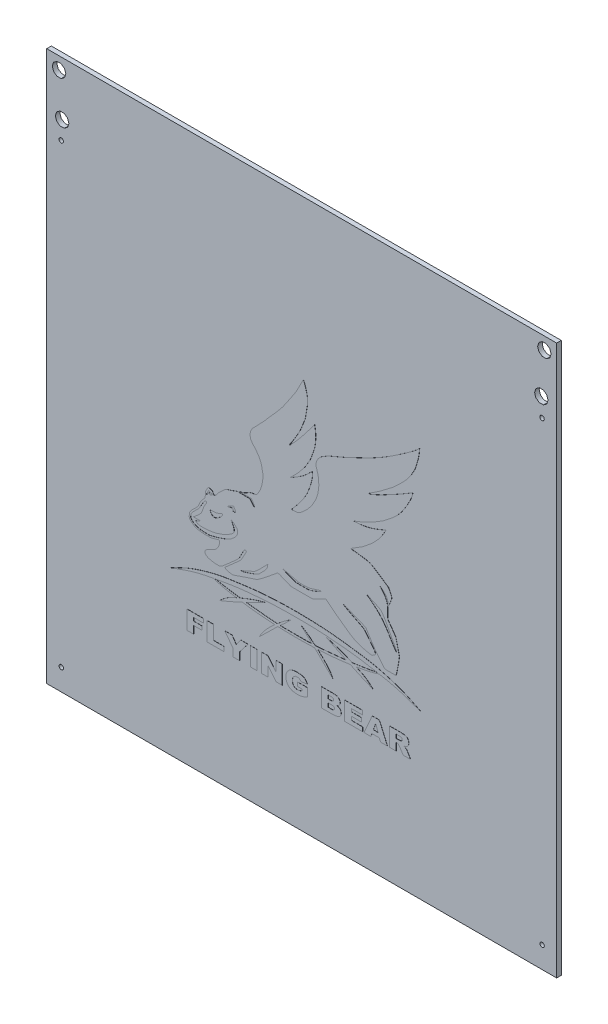
# Autodesk Inventor part: боковая  панель
Saved by Autodesk Inventor 2017 (Build 210142000, 142)
## iProperties
Part Number: боковая  панель
Material: Типовые
Document SubType Name: Modeling
Designer: Max
Mass: 356.832 g
Surface Area: 2420.3 cm^2
Volume: 356.832 cm^3
Density: 1 g/cm^3
Appearance: Чугун серый
Author: Max
Autodesk Inventor part; units mm, degrees
(part 1 of 2)
ref_plane "YZ Plane" through (0, 0, 0) normal (1, 0, 0) x (0, 1, 0)
ref_plane "XZ Plane" through (0, 0, 0) normal (0, 1, 0) x (-1, 0, 0)
ref_plane "XY Plane" through (0, 0, 0) normal (0, 0, 1) x (1, 0, 0)
sketch "Эскиз1" plane through (0, 0, 0) normal (0, 0, 1) x (1, 0, 0)
  circle A0 centre (8.5, 9) radius 1.5 projected
  circle A1 centre (8.5, 306) radius 1.5 projected
  circle A2 centre (-304.5, 306) radius 1.5 projected
  circle A3 centre (-304.5, 9) radius 1.5 projected
  line L0 (-314, 353) -> (18, 353)
  line L1 (18, 353) -> (18, -5)
  line L2 (18, -5) -> (-314, -5)
  line L3 (-314, -5) -> (-314, 353)
  circle A4 centre (10, 345) radius 4.4
  circle A5 centre (8, 318) radius 4.4
  circle A6 centre (-306, 345) radius 4.4
  circle A7 centre (-304, 318) radius 4.4
  point P0 (0, 0)
  dimension "d0" = 297
  dimension "d1" = 313
  dimension "d2" = 9.5
  dimension "d3" = 9.5
  dimension "d4" = 332
  dimension "d5" = 9.5
  dimension "d6" = 358
  dimension "d7" = 14
  dimension "d8" = 47
  dimension "d26" = 8
  dimension "d27" = 8
  dimension "d28" = 10
  dimension "d29" = 35
  dimension "d30" = 8
  dimension "d31" = 35
  dimension "d32" = 10
  dimension "d33" = 8
  dimension "d34" = 8.8
  dimension "d35" = 8.8
  dimension "d36" = 8.8
  dimension "d37" = 8.8
  constraints: 8 end point, 4 centre point, 2 parallel, 1 horizontal, 1 perpendicular
  measures "d0" distance of A0.centre A1.centre
  measures "d1" distance of A0.centre A3.centre
  measures "d2" distance from line of L1 A0.centre
  measures "d3" distance from line of L1 A1.centre
  measures "d4" distance between parallel lines of L1 L3
  measures "d5" distance from line of A3.centre L3
  measures "d6" distance between parallel lines of L0 L2
  measures "d7" distance from line of A3.centre L2
  measures "d8" distance from line of L0 A2.centre
  measures "d26" distance from line of L1 A4.centre
  measures "d27" distance from line of A4.centre L0
  measures "d28" distance from line of L1 A5.centre
  measures "d29" distance from line of L0 A5.centre
  measures "d30" distance from line of L0 A6.centre
  measures "d31" distance from line of A7.centre L0
  measures "d32" horizontal distance of L0.start A7.centre
  measures "d33" horizontal distance of A6.centre L0.start
  measures "d34" diameter of A6
  measures "d35" diameter of A7
  measures "d36" diameter of A4
  measures "d37" diameter of A5
extrude "Выдавливание1" add sketch "Эскиз1" along normal blind 3
sketch "Эскиз2" plane through (0, 0, 3) normal (0, 0, 1) x (1, 0, 0)
  line L0 (-180.2045, 205.6908) -> (-177.0361, 208.9639) construction
  line L1 (-177.0361, 208.9639) -> (-173.0672, 213.1037) construction
  line L2 (-173.0672, 213.1037) -> (-170.4432, 215.9574) construction
  line L3 (-170.4432, 215.9574) -> (-168.8687, 218.0566) construction
  line L4 (-168.8687, 218.0566) -> (-164.9525, 222.1283) construction
  line L5 (-164.9525, 222.1283) -> (-161.4603, 226.3362) construction
  line L6 (-161.4603, 226.3362) -> (-160.288, 227.7676) construction
  line L7 (-160.288, 227.7676) -> (-152.6607, 239.1023) construction
  line L8 (-152.6607, 239.1023) -> (-151.6323, 240.6673) construction
  line L9 (-151.6323, 240.6673) -> (-149.9316, 243.8361) construction
  line L10 (-149.9316, 243.8361) -> (-148.3507, 246.9727) construction
  line L11 (-148.3507, 246.9727) -> (-146.851, 249.9512) construction
  line L12 (-146.851, 249.9512) -> (-146.8254, 250.015) construction
  line L13 (-146.8254, 250.015) -> (-146.8254, 249.9575) construction
  line L14 (-146.8254, 249.9575) -> (-146.0075, 248.3799) construction
  line L15 (-146.0075, 248.3799) -> (-144.426, 243.2509) construction
  line L16 (-144.426, 243.2509) -> (-144.0276, 240.6093) construction
  line L17 (-144.0276, 240.6093) -> (-144.0276, 237.8628) construction
  line L18 (-144.0276, 237.8628) -> (-145.0701, 229.6994) construction
  line L19 (-145.0701, 229.6994) -> (-146.4307, 225.9017) construction
  line L20 (-146.4307, 225.9017) -> (-149.1507, 219.4923) construction
  line L21 (-149.1507, 219.4923) -> (-151.6499, 215.3156) construction
  line L22 (-151.6499, 215.3156) -> (-154.3887, 211.0362) construction
  line L23 (-154.3887, 211.0362) -> (-155.1076, 209.9749) construction
  line L24 (-155.1076, 209.9749) -> (-156.1304, 208.4939) construction
  line L25 (-156.1304, 208.4939) -> (-155.9009, 208.6294) construction
  line L26 (-155.9009, 208.6294) -> (-155.5783, 208.8301) construction
  line L27 (-155.5783, 208.8301) -> (-154.5963, 209.615) construction
  line L28 (-154.5963, 209.615) -> (-150.9546, 213.5612) construction
  line L29 (-150.9546, 213.5612) -> (-145.5874, 220.0786) construction
  line L30 (-145.5874, 220.0786) -> (-139.5565, 228.2444) construction
  line L31 (-139.5565, 228.2444) -> (-139.4969, 228.3364) construction
  line L32 (-139.4969, 228.3364) -> (-139.5299, 228.2418) construction
  line L33 (-139.5299, 228.2418) -> (-139.3563, 227.561) construction
  line L34 (-139.3563, 227.561) -> (-138.9367, 225.0891) construction
  line L35 (-138.9367, 225.0891) -> (-138.5378, 221.4685) construction
  line L36 (-138.5378, 221.4685) -> (-139.0937, 215.6761) construction
  line L37 (-139.0937, 215.6761) -> (-140.9097, 209.7093) construction
  line L38 (-140.9097, 209.7093) -> (-143.5781, 204.4836) construction
  line L39 (-143.5781, 204.4836) -> (-146.543, 199.8881) construction
  line L40 (-146.543, 199.8881) -> (-150.7936, 195.0629) construction
  line L41 (-150.7936, 195.0629) -> (-152.871, 193.083) construction
  line L42 (-152.871, 193.083) -> (-154.5999, 191.4239) construction
  line L43 (-154.5999, 191.4239) -> (-155.5201, 190.4339) construction
  line L44 (-155.5201, 190.4339) -> (-155.5742, 190.3528) construction
  line L45 (-155.5742, 190.3528) -> (-155.4326, 190.4314) construction
  line L46 (-155.4326, 190.4314) -> (-153.8538, 191.4333) construction
  line L47 (-153.8538, 191.4333) -> (-152.2645, 192.2568) construction
  line L48 (-152.2645, 192.2568) -> (-149.2402, 194.1507) construction
  line L49 (-149.2402, 194.1507) -> (-146.2078, 196.1384) construction
  line L50 (-146.2078, 196.1384) -> (-144.4494, 197.8457) construction
  line L51 (-144.4494, 197.8457) -> (-142.5127, 199.706) construction
  line L52 (-142.5127, 199.706) -> (-141.1876, 201.0821) construction
  line L53 (-141.1876, 201.0821) -> (-141.1211, 201.1736) construction
  line L54 (-141.1211, 201.1736) -> (-141.1521, 201.0592) construction
  line L55 (-141.1521, 201.0592) -> (-140.789, 198.921) construction
  line L56 (-140.789, 198.921) -> (-141.0832, 196.2734) construction
  line L57 (-141.0832, 196.2734) -> (-143.5783, 187.7744) construction
  line L58 (-143.5783, 187.7744) -> (-147.4823, 181.1681) construction
  line L59 (-147.4823, 181.1681) -> (-154.6365, 172.9333) construction
  line L60 (-154.6365, 172.9333) -> (-154.6413, 172.9279) construction
  line L61 (-154.6413, 172.9279) -> (-154.6261, 172.9325) construction
  line L62 (-154.6261, 172.9325) -> (-150.5488, 173.1303) construction
  line L63 (-150.5488, 173.1303) -> (-150.5023, 173.1303) construction
  line L64 (-150.5023, 173.1303) -> (-150.4241, 173.1753) construction
  line L65 (-150.4241, 173.1753) -> (-148.6376, 174.0969) construction
  line L66 (-148.6376, 174.0969) -> (-145.9899, 176.3194) construction
  line L67 (-145.9899, 176.3194) -> (-143.6414, 178.7272) construction
  line L68 (-143.6414, 178.7272) -> (-141.2139, 181.648) construction
  line L69 (-141.2139, 181.648) -> (-138.637, 186.2308) construction
  line L70 (-138.637, 186.2308) -> (-137.7784, 188.5813) construction
  line L71 (-137.7784, 188.5813) -> (-136.7423, 192.9865) construction
  line L72 (-136.7423, 192.9865) -> (-136.7423, 195.346) construction
  line L73 (-136.7423, 195.346) -> (-136.7423, 199.308) construction
  line L74 (-136.7423, 199.308) -> (-137.351, 201.832) construction
  line L75 (-137.351, 201.832) -> (-137.9585, 203.1815) construction
  line L76 (-137.9585, 203.1815) -> (-138.5823, 204.6492) construction
  line L77 (-138.5823, 204.6492) -> (-138.7474, 205.6908) construction
  line L78 (-138.7474, 205.6908) -> (-138.5929, 207.7385) construction
  line L79 (-138.5929, 207.7385) -> (-137.7581, 209.4958) construction
  line L80 (-137.7581, 209.4958) -> (-136.7322, 211.0337) construction
  line L81 (-136.7322, 211.0337) -> (-134.1061, 213.2212) construction
  line L82 (-134.1061, 213.2212) -> (-131.0548, 214.9609) construction
  line L83 (-131.0548, 214.9609) -> (-125.9426, 217.1289) construction
  line L84 (-125.9426, 217.1289) -> (-120.429, 219.2434) construction
  line L85 (-120.429, 219.2434) -> (-111.0683, 223.8533) construction
  line L86 (-111.0683, 223.8533) -> (-101.1893, 228.475) construction
  line L87 (-101.1893, 228.475) -> (-91.9176, 233.9051) construction
  line L88 (-91.9176, 233.9051) -> (-86.9496, 237.2556) construction
  line L89 (-86.9496, 237.2556) -> (-76.65, 244.2967) construction
  line L90 (-76.65, 244.2967) -> (-73.4984, 246.8715) construction
  line L91 (-73.4984, 246.8715) -> (-71.8505, 248.334) construction
  line L92 (-71.8505, 248.334) -> (-71.1089, 249.0344) construction
  line L93 (-71.1089, 249.0344) -> (-71.0317, 249.0344) construction
  line L94 (-71.0317, 249.0344) -> (-71.2255, 248.5055) construction
  line L95 (-71.2255, 248.5055) -> (-71.2255, 246.9556) construction
  line L96 (-71.2255, 246.9556) -> (-71.9453, 242.6946) construction
  line L97 (-71.9453, 242.6946) -> (-73.4931, 236.8072) construction
  line L98 (-73.4931, 236.8072) -> (-75.2923, 233.1849) construction
  line L99 (-75.2923, 233.1849) -> (-78.2429, 228.7711) construction
  line L100 (-78.2429, 228.7711) -> (-80.9056, 225.6046) construction
  line L101 (-80.9056, 225.6046) -> (-88.7168, 218.0744) construction
  line L102 (-88.7168, 218.0744) -> (-93.9004, 214.1054) construction
  line L103 (-93.9004, 214.1054) -> (-101.4492, 208.9934) construction
  line L104 (-101.4492, 208.9934) -> (-104.0858, 207.4669) construction
  line L105 (-104.0858, 207.4669) -> (-104.0858, 207.3813) construction
  line L106 (-104.0858, 207.3813) -> (-103.6066, 207.0724) construction
  line L107 (-103.6066, 207.0724) -> (-102.7892, 207.2333) construction
  line L108 (-102.7892, 207.2333) -> (-96.5868, 210.0566) construction
  line L109 (-96.5868, 210.0566) -> (-85.8931, 215.7161) construction
  line L110 (-85.8931, 215.7161) -> (-79.7646, 219.312) construction
  line L111 (-79.7646, 219.312) -> (-75.6998, 221.7509) construction
  line L112 (-75.6998, 221.7509) -> (-75.5621, 221.8387) construction
  line L113 (-75.5621, 221.8387) -> (-75.5621, 221.3223) construction
  line L114 (-75.5621, 221.3223) -> (-77.0245, 216.3152) construction
  line L115 (-77.0245, 216.3152) -> (-82.7085, 207.0734) construction
  line L116 (-82.7085, 207.0734) -> (-86.2044, 203.347) construction
  line L117 (-86.2044, 203.347) -> (-91.7733, 198.4009) construction
  line L118 (-91.7733, 198.4009) -> (-96.3023, 195.3488) construction
  line L119 (-96.3023, 195.3488) -> (-102.062, 191.8536) construction
  line L120 (-102.062, 191.8536) -> (-107.7725, 189.2445) construction
  line L121 (-107.7725, 189.2445) -> (-112.1538, 187.3246) construction
  line L122 (-112.1538, 187.3246) -> (-113.8768, 186.98) construction
  line L123 (-113.8768, 186.98) -> (-114.0125, 186.7136) construction
  line L124 (-114.0125, 186.7136) -> (-113.6533, 186.5708) construction
  line L125 (-113.6533, 186.5708) -> (-107.5747, 186.9569) construction
  line L126 (-107.5747, 186.9569) -> (-101.6244, 188.5451) construction
  line L127 (-101.6244, 188.5451) -> (-97.9782, 189.9544) construction
  line L128 (-97.9782, 189.9544) -> (-93.3535, 191.865) construction
  line L129 (-93.3535, 191.865) -> (-92.8714, 192.0615) construction
  line L130 (-92.8714, 192.0615) -> (-93.1602, 191.852) construction
  line L131 (-93.1602, 191.852) -> (-93.9679, 190.2952) construction
  line L132 (-93.9679, 190.2952) -> (-96.2883, 186.5339) construction
  line L133 (-96.2883, 186.5339) -> (-98.0685, 184.2257) construction
  line L134 (-98.0685, 184.2257) -> (-101.6348, 180.439) construction
  line L135 (-101.6348, 180.439) -> (-106.2734, 176.3065) construction
  line L136 (-106.2734, 176.3065) -> (-110.5464, 173.5515) construction
  line L137 (-110.5464, 173.5515) -> (-114.6789, 171.1058) construction
  line L138 (-114.6789, 171.1058) -> (-116.1126, 170.2062) construction
  line L139 (-116.1126, 170.2062) -> (-116.219, 170.0286) construction
  line L140 (-116.219, 170.0286) -> (-114.5586, 170.0286) construction
  line L141 (-114.5586, 170.0286) -> (-110.6732, 169.621) construction
  line L142 (-110.6732, 169.621) -> (-104.7271, 168.6199) construction
  line L143 (-104.7271, 168.6199) -> (-103.1534, 168.6199) construction
  line L144 (-103.1534, 168.6199) -> (-91.4021, 160.5335) construction
  line L145 (-91.4021, 160.5335) -> (-91.3533, 160.4774) construction
  line L146 (-91.3533, 160.4774) -> (-91.1816, 160.134) construction
  line L147 (-91.1816, 160.134) -> (-89.1661, 156.0741) construction
  line L148 (-89.1661, 156.0741) -> (-89.1661, 155.5737) construction
  line L149 (-89.1661, 155.5737) -> (-89.5681, 154.2932) construction
  line L150 (-89.5681, 154.2932) -> (-90.5395, 151.4784) construction
  line L151 (-90.5395, 151.4784) -> (-91.257, 150.209) construction
  line L152 (-91.257, 150.209) -> (-91.566, 150.1317) construction
  line L153 (-91.566, 150.1317) -> (-91.566, 150.2531) construction
  line L154 (-91.566, 150.2531) -> (-91.566, 150.7278) construction
  line L155 (-91.566, 150.7278) -> (-91.6764, 152.0082) construction
  line L156 (-91.6764, 152.0082) -> (-91.9413, 153.1783) construction
  line L157 (-91.9413, 153.1783) -> (-92.6368, 155.088) construction
  line L158 (-92.6368, 155.088) -> (-94.3256, 156.6333) construction
  line L159 (-94.3256, 156.6333) -> (-95.9262, 158.0242) construction
  line L160 (-95.9262, 158.0242) -> (-96.6768, 158.3222) construction
  line L161 (-96.6768, 158.3222) -> (-96.9749, 158.3995) construction
  line L162 (-96.9749, 158.3995) -> (-96.8701, 158.3475) construction
  line L163 (-96.8701, 158.3475) -> (-96.2956, 157.8766) construction
  line L164 (-96.2956, 157.8766) -> (-94.9273, 156.285) construction
  line L165 (-94.9273, 156.285) -> (-93.124, 153.9456) construction
  line L166 (-93.124, 153.9456) -> (-92.5148, 152.3129) construction
  line L167 (-92.5148, 152.3129) -> (-91.9299, 149.9735) construction
  line L168 (-91.9299, 149.9735) -> (-91.9299, 148.9594) construction
  line L169 (-91.9299, 148.9594) -> (-91.9299, 142.9463) construction
  line L170 (-91.9299, 142.9463) -> (-91.9299, 142.2235) construction
  line L171 (-91.9299, 142.2235) -> (-90.4742, 140.5124) construction
  line L172 (-90.4742, 140.5124) -> (-86.5347, 134.8618) construction
  line L173 (-86.5347, 134.8618) -> (-86.3052, 134.3183) construction
  line L174 (-86.3052, 134.3183) -> (-86.3052, 133.0505) construction
  line L175 (-86.3052, 133.0505) -> (-84.3022, 125.647) construction
  line L176 (-84.3022, 125.647) -> (-84.3022, 124.6994) construction
  line L177 (-84.3022, 124.6994) -> (-84.5184, 122.8172) construction
  line L178 (-84.5184, 122.8172) -> (-86.3367, 113.3336) construction
  line L179 (-86.3367, 113.3336) -> (-86.5078, 113.3336) construction
  line L180 (-86.5078, 113.3336) -> (-87.2901, 113.3336) construction
  line L181 (-87.2901, 113.3336) -> (-93.4748, 113.3336) construction
  line L182 (-93.4748, 113.3336) -> (-94.0214, 113.3336) construction
  line L183 (-94.0214, 113.3336) -> (-94.9467, 114.9961) construction
  line L184 (-94.9467, 114.9961) -> (-98.9456, 119.3916) construction
  line L185 (-98.9456, 119.3916) -> (-100.0032, 120.9448) construction
  line L186 (-100.0032, 120.9448) -> (-106.018, 130.2315) construction
  line L187 (-106.018, 130.2315) -> (-106.215, 130.694) construction
  line L188 (-106.215, 130.694) -> (-106.6783, 130.8203) construction
  line L189 (-106.6783, 130.8203) -> (-120.5865, 136.5083) construction
  line L190 (-120.5865, 136.5083) -> (-120.6842, 136.5083) construction
  line L191 (-120.6842, 136.5083) -> (-120.6842, 135.7899) construction
  line L192 (-120.6842, 135.7899) -> (-107.7997, 129.5862) construction
  line L193 (-107.7997, 129.5862) -> (-107.1982, 129.0639) construction
  line L194 (-107.1982, 129.0639) -> (-106.0151, 127.5405) construction
  line L195 (-106.0151, 127.5405) -> (-101.2131, 121.3926) construction
  line L196 (-101.2131, 121.3926) -> (-99.7156, 119.3405) construction
  line L197 (-99.7156, 119.3405) -> (-99.7156, 118.1853) construction
  line L198 (-99.7156, 118.1853) -> (-101.9371, 116.8524) construction
  line L199 (-101.9371, 116.8524) -> (-103.5365, 116.8524) construction
  line L200 (-103.5365, 116.8524) -> (-107.4464, 117.9484) construction
  line L201 (-107.4464, 117.9484) -> (-112.9293, 119.2821) construction
  line L202 (-112.9293, 119.2821) -> (-117.2673, 122.3561) construction
  line L203 (-117.2673, 122.3561) -> (-125.6526, 128.3292) construction
  line L204 (-125.6526, 128.3292) -> (-132.3149, 133.728) construction
  line L205 (-132.3149, 133.728) -> (-132.126, 133.8212) construction
  line L206 (-132.126, 133.8212) -> (-132.8175, 133.2753) construction
  line L207 (-132.8175, 133.2753) -> (-140.6236, 129.3632) construction
  line L208 (-140.6236, 129.3632) -> (-140.9553, 129.3632) construction
  line L209 (-140.9553, 129.3632) -> (-142.7265, 129.3632) construction
  line L210 (-142.7265, 129.3632) -> (-154.9526, 129.3632) construction
  line L211 (-154.9526, 129.3632) -> (-155.1733, 129.4132) construction
  line L212 (-155.1733, 129.4132) -> (-155.4392, 129.6496) construction
  line L213 (-155.4392, 129.6496) -> (-163.3327, 132.864) construction
  line L214 (-163.3327, 132.864) -> (-163.5864, 132.864) construction
  line L215 (-163.5864, 132.864) -> (-164.5688, 131.6844) construction
  line L216 (-164.5688, 131.6844) -> (-176.3163, 122.4788) construction
  line L217 (-176.3163, 122.4788) -> (-176.8534, 122.1588) construction
  line L218 (-176.8534, 122.1588) -> (-182.8586, 120.3906) construction
  line L219 (-182.8586, 120.3906) -> (-192.5336, 116.921) construction
  line L220 (-192.5336, 116.921) -> (-193.8347, 116.7208) construction
  line L221 (-193.8347, 116.7208) -> (-195.9031, 117.4548) construction
  line L222 (-195.9031, 117.4548) -> (-198.1717, 118.4556) construction
  line L223 (-198.1717, 118.4556) -> (-198.1717, 118.5559) construction
  line L224 (-198.1717, 118.5559) -> (-197.5373, 118.8968) construction
  line L225 (-197.5373, 118.8968) -> (-187.5242, 127.8743) construction
  line L226 (-187.5242, 127.8743) -> (-187.343, 127.9999) construction
  line L227 (-187.343, 127.9999) -> (-187.0311, 128.8156) construction
  line L228 (-187.0311, 128.8156) -> (-183.7764, 134.5353) construction
  line L229 (-183.7764, 134.5353) -> (-183.7764, 134.6318) construction
  line L230 (-183.7764, 134.6318) -> (-185.0783, 135.1622) construction
  line L231 (-185.0783, 135.1622) -> (-185.3677, 134.8384) construction
  line L232 (-185.3677, 134.8384) -> (-188.4981, 128.4994) construction
  line L233 (-188.4981, 128.4994) -> (-188.8328, 127.9639) construction
  line L234 (-188.8328, 127.9639) -> (-200.3103, 117.8026) construction
  line L235 (-200.3103, 117.8026) -> (-201.0177, 117.5182) construction
  line L236 (-201.0177, 117.5182) -> (-203.6469, 117.5182) construction
  line L237 (-203.6469, 117.5182) -> (-206.0855, 117.8611) construction
  line L238 (-206.0855, 117.8611) -> (-209.5599, 118.534) construction
  line L239 (-209.5599, 118.534) -> (-211.0538, 120.2854) construction
  line L240 (-211.0538, 120.2854) -> (-211.0538, 121.2384) construction
  line L241 (-211.0538, 121.2384) -> (-210.4357, 122.3717) construction
  line L242 (-210.4357, 122.3717) -> (-208.0146, 123.9686) construction
  line L243 (-208.0146, 123.9686) -> (-206.0828, 124.4322) construction
  line L244 (-206.0828, 124.4322) -> (-203.7647, 125.8231) construction
  line L245 (-203.7647, 125.8231) -> (-203.4299, 126.1837) construction
  line L246 (-203.4299, 126.1837) -> (-202.0648, 127.9351) construction
  line L247 (-202.0648, 127.9351) -> (-201.5497, 129.6865) construction
  line L248 (-201.5497, 129.6865) -> (-201.3054, 130.6523) construction
  line L249 (-201.3054, 130.6523) -> (-201.6177, 132.2504) construction
  line L250 (-201.6177, 132.2504) -> (-201.783, 132.2504) construction
  line L251 (-201.783, 132.2504) -> (-202.7749, 131.9381) construction
  line L252 (-202.7749, 131.9381) -> (-204.7771, 131.2401) construction
  line L253 (-204.7771, 131.2401) -> (-207.9548, 130.487) construction
  line L254 (-207.9548, 130.487) -> (-210.9579, 130.6932) construction
  line L255 (-210.9579, 130.6932) -> (-215.2456, 131.0336) construction
  line L256 (-215.2456, 131.0336) -> (-216.2846, 131.323) construction
  line L257 (-216.2846, 131.323) -> (-218.5042, 132.1029) construction
  line L258 (-218.5042, 132.1029) -> (-220.9938, 134.2925) construction
  line L259 (-220.9938, 134.2925) -> (-221.2338, 135.6423) construction
  line L260 (-221.2338, 135.6423) -> (-221.2338, 137.742) construction
  line L261 (-221.2338, 137.742) -> (-220.1239, 139.6916) construction
  line L262 (-220.1239, 139.6916) -> (-218.5386, 141.0887) construction
  line L263 (-218.5386, 141.0887) -> (-216.5319, 143.019) construction
  line L264 (-216.5319, 143.019) -> (-215.5189, 143.8026) construction
  line L265 (-215.5189, 143.8026) -> (-214.1688, 146.7968) construction
  line L266 (-214.1688, 146.7968) -> (-213.4971, 148.6055) construction
  line L267 (-213.4971, 148.6055) -> (-211.921, 150.0782) construction
  line L268 (-211.921, 150.0782) -> (-210.7977, 151.1461) construction
  line L269 (-210.7977, 151.1461) -> (-210.573, 151.8599) construction
  line L270 (-210.573, 151.8599) -> (-210.7321, 154.5841) construction
  line L271 (-210.7321, 154.5841) -> (-210.5325, 155.5529) construction
  line L272 (-210.5325, 155.5529) -> (-209.9889, 156.8112) construction
  line L273 (-209.9889, 156.8112) -> (-209.0662, 157.9485) construction
  line L274 (-209.0662, 157.9485) -> (-208.6799, 158.485) construction
  line L275 (-208.6799, 158.485) -> (-206.6842, 158.2275) construction
  line L276 (-206.6842, 158.2275) -> (-205.7186, 157.2833) construction
  line L277 (-205.7186, 157.2833) -> (-205.3324, 156.3176) construction
  line L278 (-205.3324, 156.3176) -> (-205.3324, 155.7812) construction
  line L279 (-205.3324, 155.7812) -> (-204.7499, 155.7812) construction
  line L280 (-204.7499, 155.7812) -> (-203.9962, 156.222) construction
  line L281 (-203.9962, 156.222) -> (-203.2597, 156.7873) construction
  line L282 (-203.2597, 156.7873) -> (-202.8979, 158.1961) construction
  line L283 (-202.8979, 158.1961) -> (-197.8496, 162.6422) construction
  line L284 (-197.8496, 162.6422) -> (-197.2244, 163.0822) construction
  line L285 (-197.2244, 163.0822) -> (-195.8581, 163.3369) construction
  line L286 (-195.8581, 163.3369) -> (-192.1429, 164.6422) construction
  line L287 (-192.1429, 164.6422) -> (-190.165, 165.3816) construction
  line L288 (-190.165, 165.3816) -> (-189.592, 165.5664) construction
  line L289 (-189.592, 165.5664) -> (-189.592, 165.4643) construction
  line L290 (-189.592, 165.4643) -> (-181.4929, 165.4643) construction
  line L291 (-181.4929, 165.4643) -> (-181.4186, 165.3756) construction
  line L292 (-181.4186, 165.3756) -> (-180.8085, 164.4859) construction
  line L293 (-180.8085, 164.4859) -> (-179.2071, 162.3253) construction
  line L294 (-179.2071, 162.3253) -> (-178.9159, 162.2122) construction
  line L295 (-178.9159, 162.2122) -> (-178.6217, 162.3643) construction
  line L296 (-178.6217, 162.3643) -> (-178.6826, 162.4252) construction
  line L297 (-178.6826, 162.4252) -> (-178.6826, 163.1963) construction
  line L298 (-178.6826, 163.1963) -> (-180.6203, 166.1181) construction
  line L299 (-180.6203, 166.1181) -> (-180.7015, 166.1181) construction
  line L300 (-180.7015, 166.1181) -> (-181.3406, 166.0572) construction
  line L301 (-181.3406, 166.0572) -> (-188.5602, 166.0572) construction
  line L302 (-188.5602, 166.0572) -> (-188.5291, 166.0841) construction
  line L303 (-188.5291, 166.0841) -> (-188.3128, 166.1085) construction
  line L304 (-188.3128, 166.1085) -> (-187.054, 166.3579) construction
  line L305 (-187.054, 166.3579) -> (-184.878, 166.9958) construction
  line L306 (-184.878, 166.9958) -> (-181.1411, 169.1807) construction
  line L307 (-181.1411, 169.1807) -> (-180.4894, 169.5066) construction
  line L308 (-180.4894, 169.5066) -> (-179.4678, 169.4127) construction
  line L309 (-179.4678, 169.4127) -> (-178.1345, 169.4425) construction
  line L310 (-178.1345, 169.4425) -> (-177.6022, 169.6366) construction
  line L311 (-177.6022, 169.6366) -> (-176.6134, 170.4786) construction
  line L312 (-176.6134, 170.4786) -> (-175.3808, 172.823) construction
  line L313 (-175.3808, 172.823) -> (-174.1929, 175.2387) construction
  line L314 (-174.1929, 175.2387) -> (-173.6413, 177.7553) construction
  line L315 (-173.6413, 177.7553) -> (-173.4172, 179.0825) construction
  line L316 (-173.4172, 179.0825) -> (-172.913, 182.4907) construction
  line L317 (-172.913, 182.4907) -> (-173.5125, 186.8632) construction
  line L318 (-173.5125, 186.8632) -> (-174.6056, 190.1425) construction
  line L319 (-174.6056, 190.1425) -> (-175.7692, 192.4698) construction
  line L320 (-175.7692, 192.4698) -> (-177.6734, 195.2202) construction
  line L321 (-177.6734, 195.2202) -> (-179.4012, 196.7718) construction
  line L322 (-179.4012, 196.7718) -> (-180.6411, 198.1746) construction
  line L323 (-180.6411, 198.1746) -> (-181.3601, 199.7249) construction
  line L324 (-181.3601, 199.7249) -> (-181.6297, 201.3426) construction
  line L325 (-181.6297, 201.3426) -> (-181.4275, 202.9153) construction
  line L326 (-181.4275, 202.9153) -> (-181.1129, 204.4206) construction
  line L327 (-181.1129, 204.4206) -> (-180.6636, 205.1396) construction
  line L328 (-180.6636, 205.1396) -> (-180.2045, 205.6908) construction
  spline S0 degree 4 poles (-180.2045, 205.6908) (-177.0361, 208.9639) (-173.0672, 213.1037) (-170.4432, 215.9574) (-168.8687, 218.0566) (-164.9525, 222.1283) (-161.4603, 226.3362) (-160.288, 227.7676) (-152.6607, 239.1023) (-151.6323, 240.6673) (-149.9316, 243.8361) (-148.3507, 246.9727) (-146.851, 249.9512) (-146.8254, 250.015) (-146.8254, 249.9575) (-146.0075, 248.3799) (-144.426, 243.2509) (-144.0276, 240.6093) (-144.0276, 237.8628) (-145.0701, 229.6994) (-146.4307, 225.9017) (-149.1507, 219.4923) (-151.6499, 215.3156) (-154.3887, 211.0362) (-155.1076, 209.9749) (-156.1304, 208.4939) (-155.9009, 208.6294) (-155.5783, 208.8301) (-154.5963, 209.615) (-150.9546, 213.5612) (-145.5874, 220.0786) (-139.5565, 228.2444) (-139.4969, 228.3364) (-139.5299, 228.2418) (-139.3563, 227.561) (-138.9367, 225.0891) (-138.5378, 221.4685) (-139.0937, 215.6761) (-140.9097, 209.7093) (-143.5781, 204.4836) (-146.543, 199.8881) (-150.7936, 195.0629) (-152.871, 193.083) (-154.5999, 191.4239) (-155.5201, 190.4339) (-155.5742, 190.3528) (-155.4326, 190.4314) (-153.8538, 191.4333) (-152.2645, 192.2568) (-149.2402, 194.1507) (-146.2078, 196.1384) (-144.4494, 197.8457) (-142.5127, 199.706) (-141.1876, 201.0821) (-141.1211, 201.1736) (-141.1521, 201.0592) (-140.789, 198.921) (-141.0832, 196.2734) (-143.5783, 187.7744) (-147.4823, 181.1681) (-154.6365, 172.9333) (-154.6413, 172.9279) (-154.6261, 172.9325) (-150.5488, 173.1303) (-150.5023, 173.1303) (-150.4241, 173.1753) (-148.6376, 174.0969) (-145.9899, 176.3194) (-143.6414, 178.7272) (-141.2139, 181.648) (-138.637, 186.2308) (-137.7784, 188.5813) (-136.7423, 192.9865) (-136.7423, 195.346) (-136.7423, 199.308) (-137.351, 201.832) (-137.9585, 203.1815) (-138.5823, 204.6492) (-138.7474, 205.6908) (-138.5929, 207.7385) (-137.7581, 209.4958) (-136.7322, 211.0337) (-134.1061, 213.2212) (-131.0548, 214.9609) (-125.9426, 217.1289) (-120.429, 219.2434) (-111.0683, 223.8533) (-101.1893, 228.475) (-91.9176, 233.9051) (-86.9496, 237.2556) (-76.65, 244.2967) (-73.4984, 246.8715) (-71.8505, 248.334) (-71.1089, 249.0344) (-71.0317, 249.0344) (-71.2255, 248.5055) (-71.2255, 246.9556) (-71.9453, 242.6946) (-73.4931, 236.8072) (-75.2923, 233.1849) (-78.2429, 228.7711) (-80.9056, 225.6046) (-88.7168, 218.0744) (-93.9004, 214.1054) (-101.4492, 208.9934) (-104.0858, 207.4669) (-104.0858, 207.3813) (-103.6066, 207.0724) (-102.7892, 207.2333) (-96.5868, 210.0566) (-85.8931, 215.7161) (-79.7646, 219.312) (-75.6998, 221.7509) (-75.5621, 221.8387) (-75.5621, 221.3223) (-77.0245, 216.3152) (-82.7085, 207.0734) (-86.2044, 203.347) (-91.7733, 198.4009) (-96.3023, 195.3488) (-102.062, 191.8536) (-107.7725, 189.2445) (-112.1538, 187.3246) (-113.8768, 186.98) (-114.0125, 186.7136) (-113.6533, 186.5708) (-107.5747, 186.9569) (-101.6244, 188.5451) (-97.9782, 189.9544) (-93.3535, 191.865) (-92.8714, 192.0615) (-93.1602, 191.852) (-93.9679, 190.2952) (-96.2883, 186.5339) (-98.0685, 184.2257) (-101.6348, 180.439) (-106.2734, 176.3065) (-110.5464, 173.5515) (-114.6789, 171.1058) (-116.1126, 170.2062) (-116.219, 170.0286) (-114.5586, 170.0286) (-110.6732, 169.621) (-104.7271, 168.6199) (-103.1534, 168.6199) (-91.4021, 160.5335) (-91.3533, 160.4774) (-91.1816, 160.134) (-89.1661, 156.0741) (-89.1661, 155.5737) (-89.5681, 154.2932) (-90.5395, 151.4784) (-91.257, 150.209) (-91.566, 150.1317) (-91.566, 150.2531) (-91.566, 150.7278) (-91.6764, 152.0082) (-91.9413, 153.1783) (-92.6368, 155.088) (-94.3256, 156.6333) (-95.9262, 158.0242) (-96.6768, 158.3222) (-96.9749, 158.3995) (-96.8701, 158.3475) (-96.2956, 157.8766) (-94.9273, 156.285) (-93.124, 153.9456) (-92.5148, 152.3129) (-91.9299, 149.9735) (-91.9299, 148.9594) (-91.9299, 142.9463) (-91.9299, 142.2235) (-90.4742, 140.5124) (-86.5347, 134.8618) (-86.3052, 134.3183) (-86.3052, 133.0505) (-84.3022, 125.647) (-84.3022, 124.6994) (-84.5184, 122.8172) (-86.3367, 113.3336) (-86.5078, 113.3336) (-87.2901, 113.3336) (-93.4748, 113.3336) (-94.0214, 113.3336) (-94.9467, 114.9961) (-98.9456, 119.3916) (-100.0032, 120.9448) (-106.018, 130.2315) (-106.215, 130.694) (-106.6783, 130.8203) (-120.5865, 136.5083) (-120.6842, 136.5083) (-120.6842, 135.7899) (-107.7997, 129.5862) (-107.1982, 129.0639) (-106.0151, 127.5405) (-101.2131, 121.3926) (-99.7156, 119.3405) (-99.7156, 118.1853) (-101.9371, 116.8524) (-103.5365, 116.8524) (-107.4464, 117.9484) (-112.9293, 119.2821) (-117.2673, 122.3561) (-125.6526, 128.3292) (-132.3149, 133.728) (-132.126, 133.8212) (-132.8175, 133.2753) (-140.6236, 129.3632) (-140.9553, 129.3632) (-142.7265, 129.3632) (-154.9526, 129.3632) (-155.1733, 129.4132) (-155.4392, 129.6496) (-163.3327, 132.864) (-163.5864, 132.864) (-164.5688, 131.6844) (-176.3163, 122.4788) (-176.8534, 122.1588) (-182.8586, 120.3906) (-192.5336, 116.921) (-193.8347, 116.7208) (-195.9031, 117.4548) (-198.1717, 118.4556) (-198.1717, 118.5559) (-197.5373, 118.8968) (-187.5242, 127.8743) (-187.343, 127.9999) (-187.0311, 128.8156) (-183.7764, 134.5353) (-183.7764, 134.6318) (-185.0783, 135.1622) (-185.3677, 134.8384) (-188.4981, 128.4994) (-188.8328, 127.9639) (-200.3103, 117.8026) (-201.0177, 117.5182) (-203.6469, 117.5182) (-206.0855, 117.8611) (-209.5599, 118.534) (-211.0538, 120.2854) (-211.0538, 121.2384) (-210.4357, 122.3717) (-208.0146, 123.9686) (-206.0828, 124.4322) (-203.7647, 125.8231) (-203.4299, 126.1837) (-202.0648, 127.9351) (-201.5497, 129.6865) (-201.3054, 130.6523) (-201.6177, 132.2504) (-201.783, 132.2504) (-202.7749, 131.9381) (-204.7771, 131.2401) (-207.9548, 130.487) (-210.9579, 130.6932) (-215.2456, 131.0336) (-216.2846, 131.323) (-218.5042, 132.1029) (-220.9938, 134.2925) (-221.2338, 135.6423) (-221.2338, 137.742) (-220.1239, 139.6916) (-218.5386, 141.0887) (-216.5319, 143.019) (-215.5189, 143.8026) (-214.1688, 146.7968) (-213.4971, 148.6055) (-211.921, 150.0782) (-210.7977, 151.1461) (-210.573, 151.8599) (-210.7321, 154.5841) (-210.5325, 155.5529) (-209.9889, 156.8112) (-209.0662, 157.9485) (-208.6799, 158.485) (-206.6842, 158.2275) (-205.7186, 157.2833) (-205.3324, 156.3176) (-205.3324, 155.7812) (-204.7499, 155.7812) (-203.9962, 156.222) (-203.2597, 156.7873) (-202.8979, 158.1961) (-197.8496, 162.6422) (-197.2244, 163.0822) (-195.8581, 163.3369) (-192.1429, 164.6422) (-190.165, 165.3816) (-189.592, 165.5664) (-189.592, 165.4643) (-181.4929, 165.4643) (-181.4186, 165.3756) (-180.8085, 164.4859) (-179.2071, 162.3253) (-178.9159, 162.2122) (-178.6217, 162.3643) (-178.6826, 162.4252) (-178.6826, 163.1963) (-180.6203, 166.1181) (-180.7015, 166.1181) (-181.3406, 166.0572) (-188.5602, 166.0572) (-188.5291, 166.0841) (-188.3128, 166.1085) (-187.054, 166.3579) (-184.878, 166.9958) (-181.1411, 169.1807) (-180.4894, 169.5066) (-179.4678, 169.4127) (-178.1345, 169.4425) (-177.6022, 169.6366) (-176.6134, 170.4786) (-175.3808, 172.823) (-174.1929, 175.2387) (-173.6413, 177.7553) (-173.4172, 179.0825) (-172.913, 182.4907) (-173.5125, 186.8632) (-174.6056, 190.1425) (-175.7692, 192.4698) (-177.6734, 195.2202) (-179.4012, 196.7718) (-180.6411, 198.1746) (-181.3601, 199.7249) (-181.6297, 201.3426) (-181.4275, 202.9153) (-181.1129, 204.4206) (-180.6636, 205.1396) (-180.2045, 205.6908) knots 1 1 1 1 1 2 3 4 5 6 7 8 9 10 11 12 13 14 15 16 17 18 19 20 21 22 23 24 25 26 27 28 29 30 31 32 33 34 35 36 37 38 39 40 41 42 43 44 45 46 47 48 49 50 51 52 53 54 55 56 57 58 59 60 61 62 63 64 65 66 67 68 69 70 71 72 73 74 75 76 77 78 79 80 81 82 83 84 85 86 87 88 89 90 91 92 93 94 95 96 97 98 99 100 101 102 103 104 105 106 107 108 109 110 111 112 113 114 115 116 117 118 119 120 121 122 123 124 125 126 127 128 129 130 131 132 133 134 135 136 137 138 139 140 141 142 143 144 145 146 147 148 149 150 151 152 153 154 155 156 157 158 159 160 161 162 163 164 165 166 167 168 169 170 171 172 173 174 175 176 177 178 179 180 181 182 183 184 185 186 187 188 189 190 191 192 193 194 195 196 197 198 199 200 201 202 203 204 205 206 207 208 209 210 211 212 213 214 215 216 217 218 219 220 221 222 223 224 225 226 227 228 229 230 231 232 233 234 235 236 237 238 239 240 241 242 243 244 245 246 247 248 249 250 251 252 253 254 255 256 257 258 259 260 261 262 263 264 265 266 267 268 269 270 271 272 273 274 275 276 277 278 279 280 281 282 283 284 285 286 287 288 289 290 291 292 293 294 295 296 297 298 299 300 301 302 303 304 305 306 307 308 309 310 311 312 313 314 315 316 317 318 319 320 321 322 323 324 325 326 327 327 327 327 327
  line L329 (-195.9901, 154.0054) -> (-194.5336, 155.0578) construction
  line L330 (-194.5336, 155.0578) -> (-193.1544, 155.5487) construction
  line L331 (-193.1544, 155.5487) -> (-192.4297, 156.0162) construction
  line L332 (-192.4297, 156.0162) -> (-192.166, 155.9532) construction
  line L333 (-192.166, 155.9532) -> (-191.979, 155.402) construction
  line L334 (-191.979, 155.402) -> (-191.1227, 154.2109) construction
  line L335 (-191.1227, 154.2109) -> (-190.8274, 153.3349) construction
  line L336 (-190.8274, 153.3349) -> (-190.7388, 152.9018) construction
  line L337 (-190.7388, 152.9018) -> (-191.0734, 152.9018) construction
  line L338 (-191.0734, 152.9018) -> (-192.294, 152.9018) construction
  line L339 (-192.294, 152.9018) -> (-192.6484, 152.9018) construction
  line L340 (-192.6484, 152.9018) -> (-192.5696, 153.4825) construction
  line L341 (-192.5696, 153.4825) -> (-192.6385, 154.0054) construction
  line L342 (-192.6385, 154.0054) -> (-192.8846, 154.5259) construction
  line L343 (-192.8846, 154.5259) -> (-193.3669, 154.5259) construction
  line L344 (-193.3669, 154.5259) -> (-194.5284, 154.3586) construction
  line L345 (-194.5284, 154.3586) -> (-195.4931, 153.8073) construction
  line L346 (-195.4931, 153.8073) -> (-195.8671, 153.64) construction
  line L347 (-195.8671, 153.64) -> (-195.9901, 153.8762) construction
  line L348 (-195.9901, 153.8762) -> (-195.9901, 154.0054) construction
  spline S1 degree 4 poles (-195.9901, 154.0054) (-194.5336, 155.0578) (-193.1544, 155.5487) (-192.4297, 156.0162) (-192.166, 155.9532) (-191.979, 155.402) (-191.1227, 154.2109) (-190.8274, 153.3349) (-190.7388, 152.9018) (-191.0734, 152.9018) (-192.294, 152.9018) (-192.6484, 152.9018) (-192.5696, 153.4825) (-192.6385, 154.0054) (-192.8846, 154.5259) (-193.3669, 154.5259) (-194.5284, 154.3586) (-195.4931, 153.8073) (-195.8671, 153.64) (-195.9901, 153.8762) (-195.9901, 154.0054) knots 1 1 1 1 1 2 3 4 5 6 7 8 9 10 11 12 13 14 15 16 17 18 18 18 18 18
  line L349 (-209.8609, 154.0054) -> (-208.9336, 155.7519) construction
  line L350 (-208.9336, 155.7519) -> (-208.6363, 156.6911) construction
  line L351 (-208.6363, 156.6911) -> (-208.3748, 156.917) construction
  line L352 (-208.3748, 156.917) -> (-207.2172, 156.437) construction
  line L353 (-207.2172, 156.437) -> (-206.8017, 155.818) construction
  line L354 (-206.8017, 155.818) -> (-206.0131, 155.6315) construction
  line L355 (-206.0131, 155.6315) -> (-206.0131, 155.428) construction
  line L356 (-206.0131, 155.428) -> (-206.3523, 155.1312) construction
  line L357 (-206.3523, 155.1312) -> (-207.1324, 154.7327) construction
  line L358 (-207.1324, 154.7327) -> (-207.5139, 154.5377) construction
  line L359 (-207.5139, 154.5377) -> (-207.6072, 154.8259) construction
  line L360 (-207.6072, 154.8259) -> (-207.5054, 155.2584) construction
  line L361 (-207.5054, 155.2584) -> (-207.7005, 155.6399) construction
  line L362 (-207.7005, 155.6399) -> (-208.0905, 155.7162) construction
  line L363 (-208.0905, 155.7162) -> (-208.4805, 155.1736) construction
  line L364 (-208.4805, 155.1736) -> (-209.0232, 154.4698) construction
  line L365 (-209.0232, 154.4698) -> (-209.32, 154.0798) construction
  line L366 (-209.32, 154.0798) -> (-209.498, 153.7576) construction
  line L367 (-209.498, 153.7576) -> (-209.7863, 153.7576) construction
  line L368 (-209.7863, 153.7576) -> (-209.8609, 154.0054) construction
  spline S2 degree 4 poles (-209.8609, 154.0054) (-208.9336, 155.7519) (-208.6363, 156.6911) (-208.3748, 156.917) (-207.2172, 156.437) (-206.8017, 155.818) (-206.0131, 155.6315) (-206.0131, 155.428) (-206.3523, 155.1312) (-207.1324, 154.7327) (-207.5139, 154.5377) (-207.6072, 154.8259) (-207.5054, 155.2584) (-207.7005, 155.6399) (-208.0905, 155.7162) (-208.4805, 155.1736) (-209.0232, 154.4698) (-209.32, 154.0798) (-209.498, 153.7576) (-209.7863, 153.7576) (-209.8609, 154.0054) knots 1 1 1 1 1 2 3 4 5 6 7 8 9 10 11 12 13 14 15 16 17 18 18 18 18 18
  line L369 (-209.7279, 149.12) -> (-209.9534, 149.7791) construction
  line L370 (-209.9534, 149.7791) -> (-210.4218, 150.074) construction
  line L371 (-210.4218, 150.074) -> (-210.9248, 149.6924) construction
  line L372 (-210.9248, 149.6924) -> (-211.7227, 148.7384) construction
  line L373 (-211.7227, 148.7384) -> (-212.8905, 146.9301) construction
  line L374 (-212.8905, 146.9301) -> (-213.6517, 145.1453) construction
  line L375 (-213.6517, 145.1453) -> (-214.4391, 143.7805) construction
  line L376 (-214.4391, 143.7805) -> (-215.489, 142.4944) construction
  line L377 (-215.489, 142.4944) -> (-216.764, 141.3837) construction
  line L378 (-216.764, 141.3837) -> (-218.4329, 140.0243) construction
  line L379 (-218.4329, 140.0243) -> (-219.8436, 138.2351) construction
  line L380 (-219.8436, 138.2351) -> (-220.2968, 137.0901) construction
  line L381 (-220.2968, 137.0901) -> (-220.2968, 136.2791) construction
  line L382 (-220.2968, 136.2791) -> (-220.1656, 135.2892) construction
  line L383 (-220.1656, 135.2892) -> (-218.9388, 133.8015) construction
  line L384 (-218.9388, 133.8015) -> (-216.8265, 132.6566) construction
  line L385 (-216.8265, 132.6566) -> (-214.4885, 131.8504) construction
  line L386 (-214.4885, 131.8504) -> (-210.6671, 131.7214) construction
  line L387 (-210.6671, 131.7214) -> (-208.2807, 131.5763) construction
  line L388 (-208.2807, 131.5763) -> (-205.7492, 132.1407) construction
  line L389 (-205.7492, 132.1407) -> (-202.9597, 132.8985) construction
  line L390 (-202.9597, 132.8985) -> (-200.3722, 133.7803) construction
  line L391 (-200.3722, 133.7803) -> (-197.1024, 134.8703) construction
  line L392 (-197.1024, 134.8703) -> (-194.5084, 136.1128) construction
  line L393 (-194.5084, 136.1128) -> (-191.0522, 138.736) construction
  line L394 (-191.0522, 138.736) -> (-190.2565, 140.4158) construction
  line L395 (-190.2565, 140.4158) -> (-189.3429, 142.0367) construction
  line L396 (-189.3429, 142.0367) -> (-189.5197, 143.1271) construction
  line L397 (-189.5197, 143.1271) -> (-189.9913, 144.5122) construction
  line L398 (-189.9913, 144.5122) -> (-190.787, 145.3669) construction
  line L399 (-190.787, 145.3669) -> (-192.4668, 146.8404) construction
  line L400 (-192.4668, 146.8404) -> (-193.4688, 147.3414) construction
  line L401 (-193.4688, 147.3414) -> (-193.9992, 147.3414) construction
  line L402 (-193.9992, 147.3414) -> (-194.2055, 147.5477) construction
  line L403 (-194.2055, 147.5477) -> (-193.233, 146.4278) construction
  line L404 (-193.233, 146.4278) -> (-192.1426, 144.6006) construction
  line L405 (-192.1426, 144.6006) -> (-191.7595, 143.1271) construction
  line L406 (-191.7595, 143.1271) -> (-191.7595, 141.2999) construction
  line L407 (-191.7595, 141.2999) -> (-192.9088, 140.0327) construction
  line L408 (-192.9088, 140.0327) -> (-195.1191, 138.5297) construction
  line L409 (-195.1191, 138.5297) -> (-200.0112, 136.0542) construction
  line L410 (-200.0112, 136.0542) -> (-204.4023, 134.6691) construction
  line L411 (-204.4023, 134.6691) -> (-209.7279, 133.9029) construction
  line L412 (-209.7279, 133.9029) -> (-214.4812, 133.9029) construction
  line L413 (-214.4812, 133.9029) -> (-216.2495, 134.5512) construction
  line L414 (-216.2495, 134.5512) -> (-217.0452, 135.1996) construction
  line L415 (-217.0452, 135.1996) -> (-217.0452, 135.5532) construction
  line L416 (-217.0452, 135.5532) -> (-216.8312, 135.3913) construction
  line L417 (-216.8312, 135.3913) -> (-216.1054, 135.6438) construction
  line L418 (-216.1054, 135.6438) -> (-215.0829, 136.0793) construction
  line L419 (-215.0829, 136.0793) -> (-214.376, 136.4138) construction
  line L420 (-214.376, 136.4138) -> (-213.9027, 136.742) construction
  line L421 (-213.9027, 136.742) -> (-213.8459, 136.8619) construction
  line L422 (-213.8459, 136.8619) -> (-213.9847, 136.8619) construction
  line L423 (-213.9847, 136.8619) -> (-218.3017, 136.8051) construction
  line L424 (-218.3017, 136.8051) -> (-218.3017, 136.9439) construction
  line L425 (-218.3017, 136.9439) -> (-218.0114, 137.2153) construction
  line L426 (-218.0114, 137.2153) -> (-217.1215, 137.8591) construction
  line L427 (-217.1215, 137.8591) -> (-214.9493, 139.8365) construction
  line L428 (-214.9493, 139.8365) -> (-213.6989, 141.0674) construction
  line L429 (-213.6989, 141.0674) -> (-212.8197, 141.9466) construction
  line L430 (-212.8197, 141.9466) -> (-212.3118, 144.0175) construction
  line L431 (-212.3118, 144.0175) -> (-211.6475, 145.9712) construction
  line L432 (-211.6475, 145.9712) -> (-211.0028, 147.2411) construction
  line L433 (-211.0028, 147.2411) -> (-210.1822, 148.3743) construction
  line L434 (-210.1822, 148.3743) -> (-209.7279, 149.12) construction
  spline S3 degree 4 poles (-209.7279, 149.12) (-209.9534, 149.7791) (-210.4218, 150.074) (-210.9248, 149.6924) (-211.7227, 148.7384) (-212.8905, 146.9301) (-213.6517, 145.1453) (-214.4391, 143.7805) (-215.489, 142.4944) (-216.764, 141.3837) (-218.4329, 140.0243) (-219.8436, 138.2351) (-220.2968, 137.0901) (-220.2968, 136.2791) (-220.1656, 135.2892) (-218.9388, 133.8015) (-216.8265, 132.6566) (-214.4885, 131.8504) (-210.6671, 131.7214) (-208.2807, 131.5763) (-205.7492, 132.1407) (-202.9597, 132.8985) (-200.3722, 133.7803) (-197.1024, 134.8703) (-194.5084, 136.1128) (-191.0522, 138.736) (-190.2565, 140.4158) (-189.3429, 142.0367) (-189.5197, 143.1271) (-189.9913, 144.5122) (-190.787, 145.3669) (-192.4668, 146.8404) (-193.4688, 147.3414) (-193.9992, 147.3414) (-194.2055, 147.5477) (-193.233, 146.4278) (-192.1426, 144.6006) (-191.7595, 143.1271) (-191.7595, 141.2999) (-192.9088, 140.0327) (-195.1191, 138.5297) (-200.0112, 136.0542) (-204.4023, 134.6691) (-209.7279, 133.9029) (-214.4812, 133.9029) (-216.2495, 134.5512) (-217.0452, 135.1996) (-217.0452, 135.5532) (-216.8312, 135.3913) (-216.1054, 135.6438) (-215.0829, 136.0793) (-214.376, 136.4138) (-213.9027, 136.742) (-213.8459, 136.8619) (-213.9847, 136.8619) (-218.3017, 136.8051) (-218.3017, 136.9439) (-218.0114, 137.2153) (-217.1215, 137.8591) (-214.9493, 139.8365) (-213.6989, 141.0674) (-212.8197, 141.9466) (-212.3118, 144.0175) (-211.6475, 145.9712) (-211.0028, 147.2411) (-210.1822, 148.3743) (-209.7279, 149.12) knots 1 1 1 1 1 2 3 4 5 6 7 8 9 10 11 12 13 14 15 16 17 18 19 20 21 22 23 24 25 26 27 28 29 30 31 32 33 34 35 36 37 38 39 40 41 42 43 44 45 46 47 48 49 50 51 52 53 54 55 56 57 58 59 60 61 62 63 64 64 64 64 64
  line L435 (-207.5871, 146.3401) -> (-204.8026, 146.3401) construction
  line L436 (-204.8026, 146.3401) -> (-202.9147, 146.5761) construction
  line L437 (-202.9147, 146.5761) -> (-201.2864, 147.3548) construction
  line L438 (-201.2864, 147.3548) -> (-200.2717, 147.756) construction
  line L439 (-200.2717, 147.756) -> (-199.1154, 148.2751) construction
  line L440 (-199.1154, 148.2751) -> (-199.3494, 147.3039) construction
  line L441 (-199.3494, 147.3039) -> (-200.2551, 145.8806) construction
  line L442 (-200.2551, 145.8806) -> (-201.6784, 144.716) construction
  line L443 (-201.6784, 144.716) -> (-203.4899, 143.5084) construction
  line L444 (-203.4899, 143.5084) -> (-204.7407, 143.1633) construction
  line L445 (-204.7407, 143.1633) -> (-205.8621, 143.5084) construction
  line L446 (-205.8621, 143.5084) -> (-206.8973, 144.3278) construction
  line L447 (-206.8973, 144.3278) -> (-207.5871, 145.4061) construction
  line L448 (-207.5871, 145.4061) -> (-207.5871, 146.3401) construction
  spline S4 degree 4 poles (-207.5871, 146.3401) (-204.8026, 146.3401) (-202.9147, 146.5761) (-201.2864, 147.3548) (-200.2717, 147.756) (-199.1154, 148.2751) (-199.3494, 147.3039) (-200.2551, 145.8806) (-201.6784, 144.716) (-203.4899, 143.5084) (-204.7407, 143.1633) (-205.8621, 143.5084) (-206.8973, 144.3278) (-207.5871, 145.4061) (-207.5871, 146.3401) knots 1 1 1 1 1 2 3 4 5 6 7 8 9 10 11 12 12 12 12 12
  line L449 (-169.8892, 134.4029) -> (-177.6098, 126.4978) construction
  line L450 (-177.6098, 126.4978) -> (-178.6248, 125.9749) construction
  line L451 (-178.6248, 125.9749) -> (-179.363, 125.7595) construction
  line L452 (-179.363, 125.7595) -> (-184.7152, 123.022) construction
  line L453 (-184.7152, 123.022) -> (-187.2067, 122.4375) construction
  line L454 (-187.2067, 122.4375) -> (-187.5758, 121.8531) construction
  line L455 (-187.5758, 121.8531) -> (-186.6821, 121.8531) construction
  line L456 (-186.6821, 121.8531) -> (-183.8991, 122.6782) construction
  line L457 (-183.8991, 122.6782) -> (-179.313, 124.2461) construction
  line L458 (-179.313, 124.2461) -> (-176.8827, 125.1477) construction
  line L459 (-176.8827, 125.1477) -> (-176.5657, 125.1477) construction
  line L460 (-176.5657, 125.1477) -> (-173.938, 127.6441) construction
  line L461 (-173.938, 127.6441) -> (-171.2393, 130.4611) construction
  line L462 (-171.2393, 130.4611) -> (-170.3398, 131.9288) construction
  line L463 (-170.3398, 131.9288) -> (-169.748, 133.4202) construction
  line L464 (-169.748, 133.4202) -> (-169.8892, 134.4029) construction
  spline S5 degree 4 poles (-169.8892, 134.4029) (-177.6098, 126.4978) (-178.6248, 125.9749) (-179.363, 125.7595) (-184.7152, 123.022) (-187.2067, 122.4375) (-187.5758, 121.8531) (-186.6821, 121.8531) (-183.8991, 122.6782) (-179.313, 124.2461) (-176.8827, 125.1477) (-176.5657, 125.1477) (-173.938, 127.6441) (-171.2393, 130.4611) (-170.3398, 131.9288) (-169.748, 133.4202) (-169.8892, 134.4029) knots 1 1 1 1 1 2 3 4 5 6 7 8 9 10 11 12 13 14 14 14 14 14
  line L465 (-161.5118, 136.9026) -> (-152.0707, 133.3502) construction
  line L466 (-152.0707, 133.3502) -> (-151.8299, 133.1815) construction
  line L467 (-151.8299, 133.1815) -> (-151.4926, 133.1815) construction
  line L468 (-151.4926, 133.1815) -> (-148.6312, 133.1815) construction
  line L469 (-148.6312, 133.1815) -> (-142.7113, 133.1815) construction
  line L470 (-142.7113, 133.1815) -> (-142.5222, 133.2847) construction
  line L471 (-142.5222, 133.2847) -> (-140.2779, 134.1462) construction
  line L472 (-140.2779, 134.1462) -> (-135.1469, 136.0651) construction
  line L473 (-135.1469, 136.0651) -> (-135.1469, 136.524) construction
  line L474 (-135.1469, 136.524) -> (-135.6892, 136.524) construction
  line L475 (-135.6892, 136.524) -> (-136.4818, 136.524) construction
  line L476 (-136.4818, 136.524) -> (-140.9036, 134.8554) construction
  line L477 (-140.9036, 134.8554) -> (-143.6568, 134.1045) construction
  line L478 (-143.6568, 134.1045) -> (-146.9524, 134.1045) construction
  line L479 (-146.9524, 134.1045) -> (-151.4576, 134.1045) construction
  line L480 (-151.4576, 134.1045) -> (-153.0011, 135.1474) construction
  line L481 (-153.0011, 135.1474) -> (-156.9224, 135.9817) construction
  line L482 (-156.9224, 135.9817) -> (-161.5118, 136.9026) construction
  spline S6 degree 4 poles (-161.5118, 136.9026) (-152.0707, 133.3502) (-151.8299, 133.1815) (-151.4926, 133.1815) (-148.6312, 133.1815) (-142.7113, 133.1815) (-142.5222, 133.2847) (-140.2779, 134.1462) (-135.1469, 136.0651) (-135.1469, 136.524) (-135.6892, 136.524) (-136.4818, 136.524) (-140.9036, 134.8554) (-143.6568, 134.1045) (-146.9524, 134.1045) (-151.4576, 134.1045) (-153.0011, 135.1474) (-156.9224, 135.9817) (-161.5118, 136.9026) knots 1 1 1 1 1 2 3 4 5 6 7 8 9 10 11 12 13 14 15 16 16 16 16 16
  line L483 (-105.7825, 149.6506) -> (-98.5638, 144.2366) construction
  line L484 (-98.5638, 144.2366) -> (-96.1387, 141.0784) construction
  line L485 (-96.1387, 141.0784) -> (-92.9242, 137.6382) construction